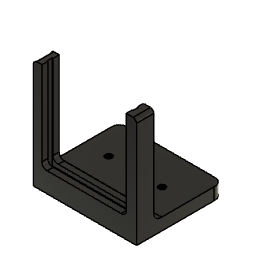
Modelo_Montura_rejilla (Autodesk Fusion 360 design; units mm, degrees)
Autodesk Fusion 360 part; units mm, degrees
sketch "Boceto1" plane through (0, 0, 0) normal (0, 1, 0) x (1, 0, 0)
  line L0 (-25, -30) -> (25, -30)
  line L1 (25, -30) -> (25, 30)
  line L2 (25, 30) -> (-25, 30)
  line L3 (-25, 30) -> (-25, -30)
  line L4 (-25, -30) -> (25, 30) construction
  line L5 (25, -30) -> (-25, 30) construction
  dimension "d1" = 50
  dimension "d2" = 60
  constraint horizontal L0
  constraint perpendicular L0 L1
  constraint parallel L0 L2
  constraint parallel L1 L3
  constraint coincident L4 origin
  constraint coincident L5 origin
  measures "d1" distance of L1.end L2.end
  measures "d2" distance of L0.end L1.end
sketch "Boceto2" plane through (0, 0, 0) normal (0, 1, 0) x (1, 0, 0)
  line L0 (30.5, -24.3703) -> (30.5, 35.6297)
  line L1 (30.5, 35.6297) -> (-29.5, 35.6297)
  line L2 (-29.5, 35.6297) -> (-29.5, -24.3703)
  line L3 (-24.5, -24.3703) -> (-24.5, 29.5)
  line L4 (-24.5, 29.5) -> (24.5, 29.5)
  line L5 (24.5, 29.5) -> (24.5, -24.3703)
  line L6 (-29.5, -24.3703) -> (-24.5, -24.3703)
  line L7 (24.5, -24.3703) -> (30.5, -24.3703)
  line L8 (25, 30) -> (-25, 30)
  line L9 (25, -30) -> (25, 30)
  line L10 (-25, 30) -> (-25, -30)
  dimension "d3" = 0.5
  dimension "d4" = 0.5
  dimension "d5" = 0.5
  constraint horizontal L6
  constraint vertical L0
  constraint horizontal L1
  constraint vertical L2
  constraint perpendicular L3 L6
  constraint perpendicular L3 L4
  constraint coincident L5.end L6
  constraint perpendicular L5 L6
  constraint collinear L6 L7
  measures "d3" distance of L4 L8
  measures "d4" distance of L5 L9
extrude "Extruir1" add sketch "Boceto2" along normal blind 5 and the other way blind 5
extrude "Extruir2" cut sketch "Boceto1" along normal blind 1.5 and the other way blind 1.5
sketch "Boceto3" plane through (0, 0, -35.6297) normal (0, 0, -1) x (1, 0, 0)
  line L0 (-29.5, 5) -> (-29.5, -5)
  line L1 (-29.5, -5) -> (30.5, -5)
  line L2 (30.5, -5) -> (30.5, 5)
  line L3 (30.5, 5) -> (-29.5, 5)
  line L4 (-29.5, 5) -> (30.5, 5)
  line L5 (30.5, 5) -> (30.5, -45)
  line L6 (30.5, -45) -> (-29.5, -45)
  line L7 (-29.5, -45) -> (-29.5, 5)
  dimension "d14" = 50
  constraint horizontal L4
  constraint vertical L5
  constraint horizontal L6
  constraint vertical L7
  constraint coincident L0.start L3.end
  constraint coincident L2.end L3.start
  measures "d14" distance of L0.start L6.end
extrude "Extruir3" add sketch "Boceto3" along normal blind 3.5 and the other way blind 3.5
fillet "Empalme1" radius 5 curvature continuous 2 edges at (30.5, 45, -35.6297) (-29.5, 45, -35.6297)
fillet "Empalme2" radius 2 curvature continuous tangency weight 0.5 2 edges at (30.5, 0, 24.3703) (-29.5, 0, 24.3703)
move_face "CarasDesfase1" offset 2 2 faces at (-8.1667, 2.6667, -29.5) (-8.1667, -3.8333, -29.5)
fillet "Empalme4" radius 4.5 curvature continuous 1 edges at (0.5, 5, -32.1297)
sketch "Boceto4" plane through (0, 0, -32.1297) normal (0, 0, 1) x (-1, 0, 0)
  line L0 (29.5, -9.5) -> (-30.5, -9.5)
  line L1 (-30.5, -9.5) -> (-30.5, -40)
  spline S0 degree 3 poles (-25.5, -45) (-26.1075, -45) (-26.7567, -45) (-27.9834, -44.6158) (-28.4633, -44.3499) (-29.3109, -43.6398) (-29.7145, -43.1816) (-30.2502, -42.1503) (-30.3672, -41.7095) (-30.5, -40.8629) (-30.5, -40.4241) (-30.5, -40) knots 0 0 0 0 0.182254 0.182254 0.32114 0.32114 0.448922 0.448922 0.55397 0.55397 0.679968 0.679968 0.679968 0.679968
  line L2 (-25.5, -45) -> (24.5, -45)
  spline S1 degree 3 poles (29.5, -40) (29.5, -40.6075) (29.5, -41.2567) (29.1158, -42.4834) (28.8499, -42.9633) (28.1398, -43.8109) (27.6816, -44.2145) (26.6503, -44.7502) (26.2095, -44.8672) (25.3629, -45) (24.9241, -45) (24.5, -45) knots 0 0 0 0 0.182254 0.182254 0.32114 0.32114 0.448922 0.448922 0.55397 0.55397 0.679968 0.679968 0.679968 0.679968
  line L3 (29.5, -40) -> (29.5, -9.5)
  line L4 (0, -2.5) -> (0, -20)
  point P0 (-15.5, -25)
  point P1 (15.5, -25)
  dimension "d28" = 15
  dimension "d29" = 20
  constraint symmetric P0 L4 P1
  measures "d28" distance of L1 P0
  measures "d29" distance of L2 P0
hole "Agujero1" at (15.5, 25, -32.1297) at (-15.5, 25, -32.1297) direction (0, 0, -1) diameter 4.5 depth 14 tip angle 180
thread "Rosca1" "ISO Metric profile 4.0 M4x0.7 6H" major diameter 4.1095 minor diameter 3.332 pitch 0.7 angle 60 modelled right hand crest width 0.193 on face at (15.6121, 22.7528, -34.463) crest through (17.166, 25, -32.3047) on face at (-15.3878, 22.7528, -34.463) crest through (-13.834, 25, -32.3047)
fillet "Empalme5" radius 3 curvature continuous 4 edges at (24.5, -3.25, -27.5) (24.5, 3.25, -27.5) (-24.5, 3.25, -27.5) (-24.5, -3.25, -27.5)
sketch "Boceto5" plane through (0, -1.5, 0) normal (0, -1, 0) x (1, 0, 0)
  line L0 (-25, 20) -> (-25, -30)
  line L1 (-25, -30) -> (25, -30)
  line L2 (25, -30) -> (25, 20)
  line L3 (25, 20) -> (-25, 20)
  line L4 (17.5, 7) -> (17.5, -16)
  line L5 (17.5, -16) -> (-17.5, -16)
  line L6 (-17.5, -16) -> (-17.5, 7)
  line L7 (-17.5, 7) -> (17.5, 7)
  point P0 (-0.25, -3.75)
  dimension "d39" = 23.75
  dimension "d40" = 24.75
  measures "d39" distance of L3 P0
  measures "d40" distance of L0 P0
equation "d39 = ( 47.5 / 2 ) * 1 mm"
equation "d40 = ( 49.5 / 2 ) * 1 mm"
